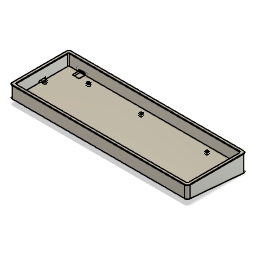
Minitomic (Autodesk Fusion 360 archive; units mm, degrees)
design "Minitomic" references "pcb"
Autodesk Fusion 360 part; units mm, degrees
sketch "Base" plane through (0, 0, 0) normal (0, 1, 0) x (1, 0, 0)
  line L0 (0, 0) -> (247, 0)
  line L1 (247, 0) -> (247, -76)
  line L2 (247, -76) -> (0, -76)
  line L3 (0, -76) -> (0, 0)
  line L4 (1.2, 0.3) -> (245.8, 0.3)
  line L5 (247.3, -1.2) -> (247.3, -74.8)
  line L6 (245.8, -76.3) -> (1.2, -76.3)
  line L7 (-0.3, -74.8) -> (-0.3, -1.2)
  line L8 (-0.8, 4.8) -> (247.8, 4.8)
  line L9 (251.8, 0.8) -> (251.8, -76.8)
  line L10 (247.8, -80.8) -> (-0.8, -80.8)
  line L11 (-4.8, -76.8) -> (-4.8, 0.8)
  arc A0 (-0.8, 4.8) -> (-4.8, 0.8) centre (-0.8, 0.8) ccw
  arc A1 (-4.8, -76.8) -> (-0.8, -80.8) centre (-0.8, -76.8) ccw
  arc A2 (247.8, -80.8) -> (251.8, -76.8) centre (247.8, -76.8) ccw
  arc A3 (251.8, 0.8) -> (247.8, 4.8) centre (247.8, 0.8) ccw
  arc A4 (247.3, -1.2) -> (245.8, 0.3) centre (245.8, -1.2) ccw
  arc A5 (245.8, -76.3) -> (247.3, -74.8) centre (245.8, -74.8) ccw
  arc A6 (-0.3, -74.8) -> (1.2, -76.3) centre (1.2, -74.8) ccw
  arc A7 (1.2, 0.3) -> (-0.3, -1.2) centre (1.2, -1.2) ccw
  dimension "d2" = 247
  dimension "d3" = 76
  dimension "d7" = 0.3
  dimension "d8" = 0.3
  dimension "d9" = 0.3
  dimension "d10" = 0.3
  dimension "d11" = 4.5
  dimension "d12" = 4.5
  dimension "d13" = 4.5
  dimension "d14" = 4.5
  dimension "d17" = 4
  dimension "d18" = 1.5
  constraint horizontal L0
  constraint vertical L1
  constraint horizontal L2
  constraint vertical L3
  constraint coincident L0.start L3.end
  constraint horizontal L4
  constraint vertical L5
  constraint horizontal L6
  constraint vertical L7
  constraint horizontal L8
  constraint vertical L9
  constraint horizontal L10
  constraint vertical L11
  constraint tangent L8 A0
  constraint tangent L11 A0
  constraint tangent L10 A1
  constraint tangent L11 A1
  constraint equal A0 A1
  constraint tangent L9 A2
  constraint tangent L10 A2
  constraint equal A0 A2
  constraint tangent L8 A3
  constraint tangent L9 A3
  constraint equal A0 A3
  constraint tangent L4 A4
  constraint tangent L5 A4
  constraint tangent L5 A5
  constraint tangent L6 A5
  constraint equal A4 A5
  constraint tangent L6 A6
  constraint tangent L7 A6
  constraint equal A4 A6
  constraint tangent L4 A7
  constraint tangent L7 A7
  constraint equal A4 A7
  measures "d2" distance of L0.start L0.end
  measures "d3" distance of L0.start L2.end
  measures "d7" distance of L0 L4
  measures "d8" distance of L3 L7
  measures "d9" distance of L2 L6
  measures "d10" distance of L1 L5
  measures "d11" distance of L5 L9
  measures "d12" distance of L6 L10
  measures "d13" distance of L7 L11
  measures "d14" distance of L4 L8
  measures "d17" radius of A0
  measures "d18" radius of A4
  measures "d57" distance of L2.end
  measures "d101" distance of L2.end
extrude "Extrude2" add sketch "Base" along normal blind 16.1 contours L0 L3 A7 | L0 L1 A4 | L2 L3 A6 | L1 L2 A5 | L8 L9 L10 L11 A0 A1 A2 A3
extrude "Extrude3" add sketch "Base" against normal blind 2 contours L0 L3 A7 | L0 L4 A4 A7 | L0 L1 L2 L3 A4 A5 A6 A7 | L3 L7 A6 A7 | L0 L1 A4 | L2 L3 A6 | L1 L5 A4 A5 | L2 L6 A5 A6 | L1 L2 A5 | L8 L9 L10 L11 A0 A1 A2 A3
sketch "Standoffs" plane through (0, 0, 0) normal (0, 1, 0) x (1, 0, 0)
  line L0 (0, 0) -> (247, 0)
  line L1 (247, 0) -> (247, -76)
  line L2 (247, -76) -> (0, -76)
  line L3 (0, -76) -> (0, 0)
  circle A0 centre (38, -9.5) radius 2.5
  circle A1 centre (38, -9.5) radius 1
  circle A2 centre (114, -9.5) radius 2.5
  circle A3 centre (114, -9.5) radius 1
  circle A4 centre (3.5, -38) radius 2.5
  circle A5 centre (3.5, -38) radius 1
  circle A6 centre (23.5, -66.5) radius 2.5
  circle A7 centre (23.5, -66.5) radius 1
  circle A8 centre (209, -9.5) radius 2.5
  circle A9 centre (209, -9.5) radius 1
  circle A10 centre (111.625, -66.5) radius 2.5
  circle A11 centre (111.625, -66.5) radius 1
  circle A12 centre (223.25, -66.5) radius 2.5
  circle A13 centre (223.25, -66.5) radius 1
  circle A14 centre (243.5, -38) radius 2.5
  circle A15 centre (243.5, -38) radius 1
  line L4 (0, 0) -> (247, 0)
  line L5 (0, -76) -> (0, 0)
  line L6 (247, 0) -> (247, -76)
  line L7 (247, -76) -> (0, -76)
  line L8 (-0.3, -35.5) -> (3.5, -35.5)
  line L9 (3.5, -35.5) -> (3.5, -40.5)
  line L10 (3.5, -40.5) -> (-0.3, -40.5)
  line L11 (-0.3, -40.5) -> (-0.3, -35.5)
  line L12 (247.3, -35.5) -> (243.5, -35.5)
  line L13 (243.5, -35.5) -> (243.5, -40.5)
  line L14 (243.5, -40.5) -> (247.3, -40.5)
  line L15 (247.3, -40.5) -> (247.3, -35.5)
  dimension "d29" = 247
  dimension "d30" = 76
  dimension "d33" = 5
  dimension "d34" = 2
  dimension "d35" = 5
  dimension "d36" = 2
  dimension "d37" = 5
  dimension "d38" = 2
  dimension "d39" = 5
  dimension "d40" = 2
  dimension "d41" = 5
  dimension "d42" = 2
  dimension "d43" = 5
  dimension "d44" = 2
  dimension "d45" = 5
  dimension "d46" = 2
  dimension "d47" = 5
  dimension "d48" = 2
  dimension "d49" = 3.5
  dimension "d50" = 38
  dimension "d51" = 38
  dimension "d52" = 9.5
  dimension "d53" = 9.5
  dimension "d54" = 114
  dimension "d55" = 38
  dimension "d56" = 9.5
  dimension "d57" = 38
  dimension "d58" = 3.5
  dimension "d59" = 9.5
  dimension "d60" = 23.5
  dimension "d61" = 9.5
  dimension "d62" = 111.625
  dimension "d63" = 223.25
  dimension "d64" = 9.5
  dimension "d70" = 0.3
  dimension "d71" = 5
  dimension "d72" = 0.3
  dimension "d73" = 5
  constraint horizontal L0
  constraint vertical L1
  constraint horizontal L2
  constraint vertical L3
  constraint coincident L0.start L3.end
  constraint concentric A0 A1
  constraint concentric A2 A3
  constraint concentric A4 A5
  constraint concentric A6 A7
  constraint concentric A8 A9
  constraint concentric A10 A11
  constraint concentric A12 A13
  constraint concentric A14 A15
  constraint horizontal L8
  constraint vertical L9
  constraint horizontal L10
  constraint vertical L11
  constraint midpoint A4.centre L9
  constraint horizontal L12
  constraint vertical L13
  constraint horizontal L14
  constraint vertical L15
  constraint midpoint A14.centre L13
  measures "d29" distance of L0.start L0.end
  measures "d30" distance of L0.start L2.end
  measures "d33" diameter of A0
  measures "d34" diameter of A1
  measures "d35" diameter of A2
  measures "d36" diameter of A3
  measures "d37" diameter of A4
  measures "d38" diameter of A5
  measures "d39" diameter of A6
  measures "d40" diameter of A7
  measures "d41" diameter of A8
  measures "d42" diameter of A9
  measures "d43" diameter of A10
  measures "d44" diameter of A11
  measures "d45" diameter of A12
  measures "d46" diameter of A13
  measures "d47" diameter of A14
  measures "d48" diameter of A15
  measures "d49" distance of L3 A4.centre
  measures "d50" distance of A4.centre L4
  measures "d51" distance of A0.centre L5
  measures "d52" distance of A0.centre L4
  measures "d53" distance of A2.centre L4
  measures "d54" distance of L3 A2.centre
  measures "d55" distance of A8.centre L6
  measures "d56" distance of A8.centre L4
  measures "d57" distance of A14.centre L4
  measures "d58" distance of A14.centre L6
  measures "d59" distance of A6.centre L7
  measures "d60" distance of L3 A6.centre
  measures "d61" distance of A10.centre L7
  measures "d62" distance of L3 A10.centre
  measures "d63" distance of A12.centre L5
  measures "d64" distance of A12.centre L7
  measures "d70" distance of L3 L11
  measures "d71" distance of L8 L10
  measures "d72" distance of L1 L15
  measures "d73" distance of L12 L14
extrude "Extrude4" add sketch "Standoffs" along normal blind 2.5 contours L3 A4 L5 L8 L10 | L3 L5 L8 L10 L11 | L1 L6 L12 L14 L15 | L1 A14 L6 L12 L14 | A4 A5 L9 | A4 A5 L9 | A14 A15 L13 | A14 A15 L13 | A0 | A2 | A6 | A8 | A10 | A12
fillet "Fillet1" radius 2 4 edges at (-0.3, 1.25, 40.5) (-0.3, 1.25, 35.5) (247.3, 1.25, 40.5) (247.3, 1.25, 35.5)
draft "Draft1" angle 5 neutral plane through (247.8, 0, 80.8) pull (0, 0, 1) 1 faces at (164.9333, -2, 52.2667)
extrude "Extrude5" cut sketch "Standoffs" against normal blind 2.5 contours A5 L9 | A5 L9 | A15 L13 | A15 L13 | A1 | A3 | A7 | A9 | A11 | A13
fillet "Fillet2" radius 0.5 16 edges at (247.3, 16.1, 38) (246.8607, 16.1, 75.8607) (123.5, 16.1, 76.3) (0.1393, 16.1, 75.8607) (-0.3, 16.1, 38) (0.1393, 16.1, 0.1393) (123.5, 16.1, -0.3) (246.8607, 16.1, 0.1393) (-4.8, 16.1, 38) (-3.6284, 16.1, 79.6284) (123.5, 16.1, 80.8) (250.6284, 16.1, 79.6284) (251.8, 16.1, 38) (250.6284, 16.1, -3.6284) (123.5, 16.1, -4.8) (-3.6284, 16.1, -3.6284)
fillet "Fillet3" radius 1 8 edges at (123.5, -9.489, -4.8) (250.6284, -9.3865, -3.6284) (251.8, -5.7445, 38) (250.6284, -2.1025, 79.6284) (123.5, -2, 80.8) (-3.6284, -2.1025, 79.6284) (-4.8, -5.7445, 38) (-3.6284, -9.3865, -3.6284)
sketch "Bumpon" plane through (0, -9.0002, 0.7874) normal (0, -0.996195, 0.087156) x (1, 0, 0)
  line L0 (-0.8, -4.5174) -> (247.8, -4.5174)
  ellipse E0 centre (247.8, -1.506) end of major axis (247.8, -4.5174) minor radius 3 (247.8, -4.5174) -> (250.8, -1.506) ccw
  line L1 (250.8, -1.506) -> (250.8, 76.3904)
  ellipse E1 centre (247.8, 76.3904) end of major axis (247.8, 79.4019) minor radius 3 (250.8, 76.3904) -> (247.8, 79.4019) ccw
  line L2 (247.8, 79.4019) -> (-0.8, 79.4019)
  ellipse E2 centre (-0.8, 76.3904) end of major axis (-0.8, 79.4019) minor radius 3 (-0.8, 79.4019) -> (-3.8, 76.3904) ccw
  line L3 (-3.8, 76.3904) -> (-3.8, -1.506)
  ellipse E3 centre (-0.8, -1.506) end of major axis (-0.8, -4.5174) minor radius 3 (-3.8, -1.506) -> (-0.8, -4.5174) ccw
  circle A0 centre (2.2, 73.3981) radius 4.05
  circle A1 centre (2.2, 1.4864) radius 4.05
  circle A2 centre (244.8, 1.4864) radius 4.05
  circle A3 centre (244.8, 73.3981) radius 4.05
  line L4 (247.8, 80.3981) -> (-0.8, 80.3981)
  line L5 (-4.8, 76.3904) -> (-4.8, -1.506)
  line L6 (-0.8, -5.5136) -> (247.8, -5.5136)
  line L7 (251.8, -1.506) -> (251.8, 76.3904)
  dimension "d82" = 8.1
  dimension "d83" = 8.1
  dimension "d84" = 8.1
  dimension "d85" = 8.1
  dimension "d86" = 7
  dimension "d89" = 7
  dimension "d90" = 7
  dimension "d91" = 7
  dimension "d92" = 7
  dimension "d93" = 7
  dimension "d94" = 7
  dimension "d95" = 7
  measures "d82" diameter of A0
  measures "d83" diameter of A1
  measures "d84" diameter of A2
  measures "d85" diameter of A3
  measures "d86" distance of A0.centre L4
  measures "d89" distance of A0.centre L5
  measures "d90" distance of A1.centre L6
  measures "d91" distance of A1.centre L5
  measures "d92" distance of A2.centre L7
  measures "d93" distance of A2.centre L6
  measures "d94" distance of A3.centre L7
  measures "d95" distance of A3.centre L4
extrude "Extrude6" cut sketch "Bumpon" against normal blind 0.5 contours A0 | A1 | A2 | A3
sketch "USB cutout" plane through (0, 0, -4.8) normal (0, 0, -1) x (-1, 0, 0)
  line L0 (-247.8, -8.3977) -> (0.8, -8.3977)
  line L1 (0.8, -8.3977) -> (0.8, 15.6)
  line L2 (0.8, 15.6) -> (-247.8, 15.6)
  line L3 (-247.8, 15.6) -> (-247.8, -8.3977)
  line L4 (-23.865, 4.875) -> (-12.865, 4.875)
  line L5 (-10.865, 2.875) -> (-10.865, -1.125)
  line L6 (-12.865, -3.125) -> (-23.865, -3.125)
  line L7 (-25.865, -1.125) -> (-25.865, 2.875)
  line L8 (-21.815, 3) -> (-14.915, 3)
  line L9 (-13.415, 1.5) -> (-13.415, 0.25)
  line L10 (-14.915, -1.25) -> (-21.815, -1.25)
  line L11 (-23.315, 0.25) -> (-23.315, 1.5)
  arc A0 (-21.815, 3) -> (-23.315, 1.5) centre (-21.815, 1.5) ccw
  arc A1 (-23.315, 0.25) -> (-21.815, -1.25) centre (-21.815, 0.25) ccw
  arc A2 (-14.915, -1.25) -> (-13.415, 0.25) centre (-14.915, 0.25) ccw
  arc A3 (-13.415, 1.5) -> (-14.915, 3) centre (-14.915, 1.5) ccw
  arc A4 (-10.865, 2.875) -> (-12.865, 4.875) centre (-12.865, 2.875) ccw
  arc A5 (-23.865, 4.875) -> (-25.865, 2.875) centre (-23.865, 2.875) ccw
  arc A6 (-25.865, -1.125) -> (-23.865, -3.125) centre (-23.865, -1.125) ccw
  arc A7 (-12.865, -3.125) -> (-10.865, -1.125) centre (-12.865, -1.125) ccw
  line L12 (4.8, -8.1353) -> (4.8, 15.6)
  line L13 (0.8, 16.1) -> (-247.8, 16.1)
  dimension "d101" = 15
  dimension "d102" = 8
  dimension "d103" = 9.9
  dimension "d104" = 4.25
  dimension "d105" = 2.55
  dimension "d106" = 1.875
  dimension "d107" = 1.5
  dimension "d108" = 2
  dimension "d109" = 15.665
  dimension "d110" = 11.225
  constraint horizontal L4
  constraint vertical L5
  constraint horizontal L6
  constraint vertical L7
  constraint horizontal L8
  constraint vertical L9
  constraint horizontal L10
  constraint vertical L11
  constraint tangent L11 A0
  constraint tangent L8 A0
  constraint tangent L10 A1
  constraint tangent L11 A1
  constraint equal A0 A1
  constraint tangent L9 A2
  constraint tangent L10 A2
  constraint equal A0 A2
  constraint tangent L8 A3
  constraint tangent L9 A3
  constraint equal A0 A3
  constraint tangent L4 A4
  constraint tangent L5 A4
  constraint tangent L4 A5
  constraint tangent L7 A5
  constraint equal A4 A5
  constraint tangent L6 A6
  constraint tangent L7 A6
  constraint equal A4 A6
  constraint tangent L5 A7
  constraint tangent L6 A7
  constraint equal A4 A7
  measures "d101" distance of L5 L7
  measures "d102" distance of L4 L6
  measures "d103" distance of L9 L11
  measures "d104" distance of L8 L10
  measures "d105" distance of L7 L11
  measures "d106" distance of L4 L8
  measures "d107" radius of A0
  measures "d108" radius of A4
  measures "d109" distance of L5 L12
  measures "d110" distance of L4 L13
extrude "Extrude7" cut sketch "USB cutout" against normal blind 3.5 contours L4 L5 L6 L7 A4 A5 A6 A7
extrude "Extrude8" cut 1 faces at (19.515, 1.5833, -4.8) along direction (0, 0, 1) blind 13
equation "u = 19 mm"
equation "d2 = 13 * u"
equation "d3 = 4 * u"
equation "keycapGap = 0.3 mm"
equation "bezel = 4.5 mm"
equation "distanceFromPlate = 7 mm"
equation "d7 = keycapGap"
equation "d8 = keycapGap"
equation "d9 = keycapGap"
equation "d10 = keycapGap"
equation "d11 = bezel"
equation "d12 = bezel"
equation "d13 = bezel"
equation "d14 = bezel"
equation "caseFillet = 4 mm"
equation "keycapFillet = 1.5 mm"
equation "d17 = caseFillet"
equation "d18 = keycapFillet"
equation "topFillet = 0.5 mm"
equation "bottomThickness = 2 mm"
equation "angle = 5 deg"
equation "standoffHeight = 2.5 mm"
equation "d25 = standoffHeight + 1.6 mm + 5 mm + distanceFromPlate"
equation "d27 = -bottomThickness"
equation "d29 = 13 * u"
equation "d30 = 4 * u"
equation "standoffDiameter = 5 mm"
equation "standoffScrewSize = 2 mm"
equation "d33 = standoffDiameter"
equation "d34 = standoffScrewSize"
equation "d35 = standoffDiameter"
equation "d36 = standoffScrewSize"
equation "d37 = standoffDiameter"
equation "d38 = standoffScrewSize"
equation "d39 = standoffDiameter"
equation "d40 = standoffScrewSize"
equation "d41 = standoffDiameter"
equation "d42 = standoffScrewSize"
equation "d43 = standoffDiameter"
equation "d44 = standoffScrewSize"
equation "d45 = standoffDiameter"
equation "d46 = standoffScrewSize"
equation "d47 = standoffDiameter"
equation "d48 = standoffScrewSize"
equation "d50 = 2 * u"
equation "d51 = 2 * u"
equation "d52 = u / 2"
equation "d53 = u / 2"
equation "d54 = 6 * u"
equation "d55 = 2 * u"
equation "d56 = u / 2"
equation "d57 = 2 * u"
equation "d59 = u / 2"
equation "d61 = u / 2"
equation "d64 = u / 2"
equation "d65 = standoffHeight"
equation "standoffScrewDepth = 5 mm"
equation "d68 = standoffHeight - standoffScrewDepth"
equation "d70 = keycapGap"
equation "d71 = standoffDiameter"
equation "d72 = keycapGap"
equation "d73 = standoffDiameter"
equation "d74 = standoffSideFillet"
equation "standoffSideFillet = 2 mm"
equation "d76 = angle"
equation "d78 = topFillet"
equation "bottomFillet = 1 mm"
equation "d80 = bottomFillet"
equation "bumponDiameter = 8.1 mm"
equation "d82 = bumponDiameter"
equation "d83 = bumponDiameter"
equation "d84 = bumponDiameter"
equation "d85 = bumponDiameter"
equation "d86 = bumponDistance"
equation "bumponDistance = 7 mm"
equation "bumponDepth = 0.5 mm"
equation "d89 = bumponDistance"
equation "d90 = bumponDistance"
equation "d91 = bumponDistance"
equation "d92 = bumponDistance"
equation "d93 = bumponDistance"
equation "d94 = bumponDistance"
equation "d95 = bumponDistance"
equation "d96 = -bumponDepth"
equation "usbCutoutPadding = 0.5 mm"
equation "usbCutoutHeight = 8 mm"
equation "usbCutoutWidth = 15 mm"
equation "d101 = usbCutoutWidth"
equation "d102 = usbCutoutHeight"
equation "d103 = 8.9 mm + usbCutoutPadding * 2"
equation "d104 = 3.25 mm + usbCutoutPadding * 2"
equation "d105 = usbCutoutWidth / 2 - d103 / 2"
equation "d106 = usbCutoutHeight / 2 - d104 / 2"
equation "d109 = bezel + keycapGap + 18.365 mm - usbCutoutWidth / 2"
equation "d110 = distanceFromPlate + 5 mm + 1.6 mm + ( ( 3.25 / 2 ) * 1 mm ) - usbCutoutHeight / 2"
equation "d111 = -bezel + 1 mm"
equation "d113 = -bezel - 8.5 mm"
named bodies: "Case"
